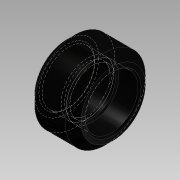
# Autodesk Inventor part: Micro V Wheel
Saved by Autodesk Inventor 2015 (Build 190159000, 159)
## iProperties
Created: 2013-06-20
Part Number: Micro V Wheel
Material: Acetal Resin, Black
Document SubType Name: Modeling
Designer: Jon Hollander
Density: 1.425 g/cm^3
Mass: 1.18321 g
Surface Area: 8.38334 cm^2
Volume: 0.830324 cm^3
Appearance: Smooth - Black
Author: Jon Hollander
Autodesk Inventor part; units mm, degrees
ref_plane "YZ Plane" through (0, 0, 0) normal (1, 0, 0) x (0, 1, 0)
ref_plane "XZ Plane" through (0, 0, 0) normal (0, 1, 0) x (-1, 0, 0)
ref_plane "XY Plane" through (0, 0, 0) normal (0, 0, 1) x (1, 0, 0)
sketch "Sketch1" plane through (0, 0, 0) normal (0, 0, 1) x (1, 0, 0)
  line L0 (0, 0) -> (5, 0)
  line L1 (0, 0) -> (0, 20) construction
  line L2 (0, 0) -> (20, 0) construction
  line L3 (0, 4.32) -> (0.5, 4.32)
  line L4 (0.5, 4.32) -> (0.5, 4.987)
  line L5 (0.5, 4.987) -> (4.1, 4.987)
  line L6 (4.4, 5.287) -> (4.4, 6.105)
  line L7 (4.4, 6.105) -> (2.89, 7.615)
  line L8 (2.89, 7.615) -> (0, 7.615)
  line L9 (4.1, 4.987) -> (4.4, 5.287)
  line L10 (0, 4.32) -> (-0.5, 4.32)
  line L11 (-0.5, 4.32) -> (-0.5, 4.987)
  line L12 (-0.5, 4.987) -> (-4.1, 4.987)
  line L13 (-4.4, 5.287) -> (-4.4, 6.105)
  line L14 (-4.4, 6.105) -> (-2.89, 7.615)
  line L15 (-2.89, 7.615) -> (0, 7.615)
  line L16 (-4.1, 4.987) -> (-4.4, 5.287)
  point P0 (4.4, 4.987)
  point P1 (-4.4, 4.987)
  dimension "d0" = 5
  dimension "d1" = 20
  dimension "d2" = 90
  dimension "d3" = 8.64
  dimension "d4" = 15.23
  dimension "d5" = 0.5
  dimension "d6" = 3.9
  dimension "d7" = 12.21
  dimension "d8" = 9.974
  dimension "d9" = 135
  dimension "d10" = 0.3
  dimension "d11" = 0.3
  dimension "d12" = 5.78
  constraints: 34 end point, 7 symmetric about line, 6 point on line, 4 perpendicular, 3 parallel, 2 horizontal
  measures "d0" distance of L0.start L0.end
  measures "d1" distance of L0.start L1.end
  measures "d2" angle of L2 L1
  measures "d3" diameter of L3 L0
  measures "d4" diameter of L8 L0
  measures "d5" distance of L3.start L3.end
  measures "d6" distance between parallel lines of L4 L6
  measures "d7" diameter of L6.end L0
  measures "d8" diameter of L5 L0
  measures "d9" angle of L6 L7
  measures "d10" distance of L5.end point (4.4, 4.987)
  measures "d11" distance of L6.start point (4.4, 4.987)
  measures "d12" distance of L15.start L7.end
revolve "Revolution1" add sketch "Sketch1" angle 360 about axis through (0, 0, 0) along (1, 0, 0)
equation "\"d11\" = d10"
body "Solid1"
